Autodesk Inventor part; units mm, degrees
(part 13 of 15)
  arc A5791 (-48.3815, -55.2875) -> (-47.8186, -55.6125) centre (-48.1, -55.45) ccw
  arc A5792 (-47.8186, -55.6125) -> (-48.3815, -55.2875) centre (-48.1, -55.45) ccw
  arc A5793 (-48.3815, -55.2875) -> (-47.8186, -55.6125) centre (-48.1, -55.45) ccw
  arc A5794 (-49.6056, -55.4035) -> (-50.1685, -55.0785) centre (-49.887, -55.241) ccw
  arc A5795 (-50.1685, -55.0785) -> (-49.6056, -55.4035) centre (-49.887, -55.241) ccw
  arc A5796 (-49.6056, -55.4035) -> (-50.1685, -55.0785) centre (-49.887, -55.241) ccw
  arc A5797 (-50.1685, -55.0785) -> (-49.6056, -55.4035) centre (-49.887, -55.241) ccw
  arc A5798 (-51.2966, -54.7885) -> (-51.8595, -54.4635) centre (-51.578, -54.626) ccw
  arc A5799 (-51.8595, -54.4635) -> (-51.2966, -54.7885) centre (-51.578, -54.626) ccw
  arc A5800 (-51.2966, -54.7885) -> (-51.8595, -54.4635) centre (-51.578, -54.626) ccw
  arc A5801 (-51.8595, -54.4635) -> (-51.2966, -54.7885) centre (-51.578, -54.626) ccw
  arc A5802 (-52.8006, -53.7995) -> (-53.3635, -53.4745) centre (-53.082, -53.637) ccw
  arc A5803 (-53.3635, -53.4745) -> (-52.8006, -53.7995) centre (-53.082, -53.637) ccw
  arc A5804 (-52.8006, -53.7995) -> (-53.3635, -53.4745) centre (-53.082, -53.637) ccw
  arc A5805 (-53.3635, -53.4745) -> (-52.8006, -53.7995) centre (-53.082, -53.637) ccw
  arc A5806 (-54.0346, -52.4905) -> (-54.5975, -52.1655) centre (-54.316, -52.328) ccw
  arc A5807 (-54.5975, -52.1655) -> (-54.0346, -52.4905) centre (-54.316, -52.328) ccw
  arc A5808 (-54.0346, -52.4905) -> (-54.5975, -52.1655) centre (-54.316, -52.328) ccw
  arc A5809 (-54.5975, -52.1655) -> (-54.0346, -52.4905) centre (-54.316, -52.328) ccw
  arc A5810 (-54.9346, -50.9325) -> (-55.4975, -50.6075) centre (-55.216, -50.77) ccw
  arc A5811 (-55.4975, -50.6075) -> (-54.9346, -50.9325) centre (-55.216, -50.77) ccw
  arc A5812 (-54.9346, -50.9325) -> (-55.4975, -50.6075) centre (-55.216, -50.77) ccw
  arc A5813 (-55.4975, -50.6075) -> (-54.9346, -50.9325) centre (-55.216, -50.77) ccw
  arc A5814 (-55.4506, -49.2085) -> (-56.0135, -48.8835) centre (-55.732, -49.046) ccw
  arc A5815 (-56.0135, -48.8835) -> (-55.4506, -49.2085) centre (-55.732, -49.046) ccw
  arc A5816 (-55.4506, -49.2085) -> (-56.0135, -48.8835) centre (-55.732, -49.046) ccw
  arc A5817 (-56.0135, -48.8835) -> (-55.4506, -49.2085) centre (-55.732, -49.046) ccw
  arc A5818 (-55.5556, -47.4115) -> (-56.1185, -47.0865) centre (-55.837, -47.249) ccw
  arc A5819 (-56.1185, -47.0865) -> (-55.5556, -47.4115) centre (-55.837, -47.249) ccw
  arc A5820 (-55.5556, -47.4115) -> (-56.1185, -47.0865) centre (-55.837, -47.249) ccw
  arc A5821 (-56.1185, -47.0865) -> (-55.5556, -47.4115) centre (-55.837, -47.249) ccw
  arc A5822 (-55.2426, -45.6395) -> (-55.8055, -45.3145) centre (-55.524, -45.477) ccw
  arc A5823 (-55.8055, -45.3145) -> (-55.2426, -45.6395) centre (-55.524, -45.477) ccw
  arc A5824 (-55.2426, -45.6395) -> (-55.8055, -45.3145) centre (-55.524, -45.477) ccw
  arc A5825 (-55.8055, -45.3145) -> (-55.2426, -45.6395) centre (-55.524, -45.477) ccw
  arc A5826 (-54.5306, -43.9875) -> (-55.0935, -43.6625) centre (-54.812, -43.825) ccw
  arc A5827 (-55.0935, -43.6625) -> (-54.5306, -43.9875) centre (-54.812, -43.825) ccw
  arc A5828 (-54.5306, -43.9875) -> (-55.0935, -43.6625) centre (-54.812, -43.825) ccw
  arc A5829 (-55.0935, -43.6625) -> (-54.5306, -43.9875) centre (-54.812, -43.825) ccw
  arc A5830 (-53.4556, -42.5445) -> (-54.0185, -42.2195) centre (-53.737, -42.382) ccw
  arc A5831 (-54.0185, -42.2195) -> (-53.4556, -42.5445) centre (-53.737, -42.382) ccw
  arc A5832 (-53.4556, -42.5445) -> (-54.0185, -42.2195) centre (-53.737, -42.382) ccw
  arc A5833 (-54.0185, -42.2195) -> (-53.4556, -42.5445) centre (-53.737, -42.382) ccw
  arc A5834 (-52.0776, -41.3875) -> (-52.6405, -41.0625) centre (-52.359, -41.225) ccw
  arc A5835 (-52.6405, -41.0625) -> (-52.0776, -41.3875) centre (-52.359, -41.225) ccw
  arc A5836 (-52.0776, -41.3875) -> (-52.6405, -41.0625) centre (-52.359, -41.225) ccw
  arc A5837 (-52.6405, -41.0625) -> (-52.0776, -41.3875) centre (-52.359, -41.225) ccw
  arc A5838 (-50.4696, -40.5795) -> (-51.0325, -40.2545) centre (-50.751, -40.417) ccw
  arc A5839 (-51.0325, -40.2545) -> (-50.4696, -40.5795) centre (-50.751, -40.417) ccw
  arc A5840 (-50.4696, -40.5795) -> (-51.0325, -40.2545) centre (-50.751, -40.417) ccw
  arc A5841 (-51.0325, -40.2545) -> (-50.4696, -40.5795) centre (-50.751, -40.417) ccw
  arc A5842 (-48.7186, -40.1645) -> (-49.2815, -39.8395) centre (-49, -40.002) ccw
  arc A5843 (-49.2815, -39.8395) -> (-48.7186, -40.1645) centre (-49, -40.002) ccw
  arc A5844 (-48.7186, -40.1645) -> (-49.2815, -39.8395) centre (-49, -40.002) ccw
  arc A5845 (-49.2815, -39.8395) -> (-48.7186, -40.1645) centre (-49, -40.002) ccw
  arc A5846 (-46.8996, -42.0595) -> (-47.4625, -41.7345) centre (-47.181, -41.897) ccw
  arc A5847 (-47.4625, -41.7345) -> (-46.8996, -42.0595) centre (-47.181, -41.897) ccw
  arc A5848 (-46.8996, -42.0595) -> (-47.4625, -41.7345) centre (-47.181, -41.897) ccw
  arc A5849 (-47.4625, -41.7345) -> (-46.8996, -42.0595) centre (-47.181, -41.897) ccw
  arc A5850 (-45.1516, -42.6275) -> (-45.7145, -42.3025) centre (-45.433, -42.465) ccw
  arc A5851 (-45.7145, -42.3025) -> (-45.1516, -42.6275) centre (-45.433, -42.465) ccw
  arc A5852 (-45.1516, -42.6275) -> (-45.7145, -42.3025) centre (-45.433, -42.465) ccw
  arc A5853 (-45.7145, -42.3025) -> (-45.1516, -42.6275) centre (-45.433, -42.465) ccw
  arc A5854 (-43.6646, -43.7085) -> (-44.2275, -43.3835) centre (-43.946, -43.546) ccw
  arc A5855 (-44.2275, -43.3835) -> (-43.6646, -43.7085) centre (-43.946, -43.546) ccw
  arc A5856 (-43.6646, -43.7085) -> (-44.2275, -43.3835) centre (-43.946, -43.546) ccw
  arc A5857 (-44.2275, -43.3835) -> (-43.6646, -43.7085) centre (-43.946, -43.546) ccw
  arc A5858 (-42.5836, -45.1955) -> (-43.1465, -44.8705) centre (-42.865, -45.033) ccw
  arc A5859 (-43.1465, -44.8705) -> (-42.5836, -45.1955) centre (-42.865, -45.033) ccw
  arc A5860 (-42.5836, -45.1955) -> (-43.1465, -44.8705) centre (-42.865, -45.033) ccw
  arc A5861 (-43.1465, -44.8705) -> (-42.5836, -45.1955) centre (-42.865, -45.033) ccw
  arc A5862 (-42.0156, -46.9435) -> (-42.5785, -46.6185) centre (-42.297, -46.781) ccw
  arc A5863 (-42.5785, -46.6185) -> (-42.0156, -46.9435) centre (-42.297, -46.781) ccw
  arc A5864 (-42.0156, -46.9435) -> (-42.5785, -46.6185) centre (-42.297, -46.781) ccw
  arc A5865 (-42.5785, -46.6185) -> (-42.0156, -46.9435) centre (-42.297, -46.781) ccw
  arc A5866 (-42.0156, -48.7815) -> (-42.5785, -48.4565) centre (-42.297, -48.619) ccw
  arc A5867 (-42.5785, -48.4565) -> (-42.0156, -48.7815) centre (-42.297, -48.619) ccw
  arc A5868 (-42.0156, -48.7815) -> (-42.5785, -48.4565) centre (-42.297, -48.619) ccw
  arc A5869 (-42.5785, -48.4565) -> (-42.0156, -48.7815) centre (-42.297, -48.619) ccw
  arc A5870 (-42.5836, -50.5295) -> (-43.1465, -50.2045) centre (-42.865, -50.367) ccw
  arc A5871 (-43.1465, -50.2045) -> (-42.5836, -50.5295) centre (-42.865, -50.367) ccw
  arc A5872 (-42.5836, -50.5295) -> (-43.1465, -50.2045) centre (-42.865, -50.367) ccw
  arc A5873 (-43.1465, -50.2045) -> (-42.5836, -50.5295) centre (-42.865, -50.367) ccw
  arc A5874 (-43.6646, -52.0165) -> (-44.2275, -51.6915) centre (-43.946, -51.854) ccw
  arc A5875 (-44.2275, -51.6915) -> (-43.6646, -52.0165) centre (-43.946, -51.854) ccw
  arc A5876 (-43.6646, -52.0165) -> (-44.2275, -51.6915) centre (-43.946, -51.854) ccw
  arc A5877 (-44.2275, -51.6915) -> (-43.6646, -52.0165) centre (-43.946, -51.854) ccw
  arc A5878 (-45.1516, -53.0975) -> (-45.7145, -52.7725) centre (-45.433, -52.935) ccw
  arc A5879 (-45.7145, -52.7725) -> (-45.1516, -53.0975) centre (-45.433, -52.935) ccw
  arc A5880 (-45.1516, -53.0975) -> (-45.7145, -52.7725) centre (-45.433, -52.935) ccw
  arc A5881 (-45.7145, -52.7725) -> (-45.1516, -53.0975) centre (-45.433, -52.935) ccw
  arc A5882 (-46.8996, -53.6655) -> (-47.4625, -53.3405) centre (-47.181, -53.503) ccw
  arc A5883 (-47.4625, -53.3405) -> (-46.8996, -53.6655) centre (-47.181, -53.503) ccw
  arc A5884 (-46.8996, -53.6655) -> (-47.4625, -53.3405) centre (-47.181, -53.503) ccw
  arc A5885 (-47.4625, -53.3405) -> (-46.8996, -53.6655) centre (-47.181, -53.503) ccw
  arc A5886 (-48.7376, -53.6655) -> (-49.3005, -53.3405) centre (-49.019, -53.503) ccw
  arc A5887 (-49.3005, -53.3405) -> (-48.7376, -53.6655) centre (-49.019, -53.503) ccw
  arc A5888 (-48.7376, -53.6655) -> (-49.3005, -53.3405) centre (-49.019, -53.503) ccw
  arc A5889 (-49.3005, -53.3405) -> (-48.7376, -53.6655) centre (-49.019, -53.503) ccw
  arc A5890 (-50.4856, -53.0975) -> (-51.0485, -52.7725) centre (-50.767, -52.935) ccw
  arc A5891 (-51.0485, -52.7725) -> (-50.4856, -53.0975) centre (-50.767, -52.935) ccw
  arc A5892 (-50.4856, -53.0975) -> (-51.0485, -52.7725) centre (-50.767, -52.935) ccw
  arc A5893 (-51.0485, -52.7725) -> (-50.4856, -53.0975) centre (-50.767, -52.935) ccw
  arc A5894 (-51.9726, -52.0165) -> (-52.5355, -51.6915) centre (-52.254, -51.854) ccw
  arc A5895 (-52.5355, -51.6915) -> (-51.9726, -52.0165) centre (-52.254, -51.854) ccw
  arc A5896 (-51.9726, -52.0165) -> (-52.5355, -51.6915) centre (-52.254, -51.854) ccw
  arc A5897 (-52.5355, -51.6915) -> (-51.9726, -52.0165) centre (-52.254, -51.854) ccw
  arc A5898 (-53.0536, -50.5295) -> (-53.6165, -50.2045) centre (-53.335, -50.367) ccw
  arc A5899 (-53.6165, -50.2045) -> (-53.0536, -50.5295) centre (-53.335, -50.367) ccw
  arc A5900 (-53.0536, -50.5295) -> (-53.6165, -50.2045) centre (-53.335, -50.367) ccw
  arc A5901 (-53.6165, -50.2045) -> (-53.0536, -50.5295) centre (-53.335, -50.367) ccw
  arc A5902 (-53.6216, -48.7815) -> (-54.1845, -48.4565) centre (-53.903, -48.619) ccw
  arc A5903 (-54.1845, -48.4565) -> (-53.6216, -48.7815) centre (-53.903, -48.619) ccw
  arc A5904 (-53.6216, -48.7815) -> (-54.1845, -48.4565) centre (-53.903, -48.619) ccw
  arc A5905 (-54.1845, -48.4565) -> (-53.6216, -48.7815) centre (-53.903, -48.619) ccw
  arc A5906 (-53.6216, -46.9435) -> (-54.1845, -46.6185) centre (-53.903, -46.781) ccw
  arc A5907 (-54.1845, -46.6185) -> (-53.6216, -46.9435) centre (-53.903, -46.781) ccw
  arc A5908 (-53.6216, -46.9435) -> (-54.1845, -46.6185) centre (-53.903, -46.781) ccw
  arc A5909 (-54.1845, -46.6185) -> (-53.6216, -46.9435) centre (-53.903, -46.781) ccw
  arc A5910 (-53.0536, -45.1955) -> (-53.6165, -44.8705) centre (-53.335, -45.033) ccw
  arc A5911 (-53.6165, -44.8705) -> (-53.0536, -45.1955) centre (-53.335, -45.033) ccw
  arc A5912 (-53.0536, -45.1955) -> (-53.6165, -44.8705) centre (-53.335, -45.033) ccw
  arc A5913 (-53.6165, -44.8705) -> (-53.0536, -45.1955) centre (-53.335, -45.033) ccw
  arc A5914 (-51.9726, -43.7085) -> (-52.5355, -43.3835) centre (-52.254, -43.546) ccw
  arc A5915 (-52.5355, -43.3835) -> (-51.9726, -43.7085) centre (-52.254, -43.546) ccw
  arc A5916 (-51.9726, -43.7085) -> (-52.5355, -43.3835) centre (-52.254, -43.546) ccw
  arc A5917 (-52.5355, -43.3835) -> (-51.9726, -43.7085) centre (-52.254, -43.546) ccw
  arc A5918 (-50.4856, -42.6275) -> (-51.0485, -42.3025) centre (-50.767, -42.465) ccw
  arc A5919 (-51.0485, -42.3025) -> (-50.4856, -42.6275) centre (-50.767, -42.465) ccw
  arc A5920 (-50.4856, -42.6275) -> (-51.0485, -42.3025) centre (-50.767, -42.465) ccw
  arc A5921 (-51.0485, -42.3025) -> (-50.4856, -42.6275) centre (-50.767, -42.465) ccw
  arc A5922 (-48.7376, -42.0595) -> (-49.3005, -41.7345) centre (-49.019, -41.897) ccw
  arc A5923 (-49.3005, -41.7345) -> (-48.7376, -42.0595) centre (-49.019, -41.897) ccw
  arc A5924 (-48.7376, -42.0595) -> (-49.3005, -41.7345) centre (-49.019, -41.897) ccw
  arc A5925 (-49.3005, -41.7345) -> (-48.7376, -42.0595) centre (-49.019, -41.897) ccw
  arc A5926 (-46.8616, -43.9785) -> (-47.4245, -43.6535) centre (-47.143, -43.816) ccw
  arc A5927 (-47.4245, -43.6535) -> (-46.8616, -43.9785) centre (-47.143, -43.816) ccw
  arc A5928 (-46.8616, -43.9785) -> (-47.4245, -43.6535) centre (-47.143, -43.816) ccw
  arc A5929 (-47.4245, -43.6535) -> (-46.8616, -43.9785) centre (-47.143, -43.816) ccw
  arc A5930 (-45.1666, -44.8685) -> (-45.7295, -44.5435) centre (-45.448, -44.706) ccw
  arc A5931 (-45.7295, -44.5435) -> (-45.1666, -44.8685) centre (-45.448, -44.706) ccw
  arc A5932 (-45.1666, -44.8685) -> (-45.7295, -44.5435) centre (-45.448, -44.706) ccw
  arc A5933 (-45.7295, -44.5435) -> (-45.1666, -44.8685) centre (-45.448, -44.706) ccw
  arc A5934 (-44.0786, -46.4445) -> (-44.6415, -46.1195) centre (-44.36, -46.282) ccw
  arc A5935 (-44.6415, -46.1195) -> (-44.0786, -46.4445) centre (-44.36, -46.282) ccw
  arc A5936 (-44.0786, -46.4445) -> (-44.6415, -46.1195) centre (-44.36, -46.282) ccw
  arc A5937 (-44.6415, -46.1195) -> (-44.0786, -46.4445) centre (-44.36, -46.282) ccw
  arc A5938 (-43.8476, -48.3445) -> (-44.4105, -48.0195) centre (-44.129, -48.182) ccw
  arc A5939 (-44.4105, -48.0195) -> (-43.8476, -48.3445) centre (-44.129, -48.182) ccw
  arc A5940 (-43.8476, -48.3445) -> (-44.4105, -48.0195) centre (-44.129, -48.182) ccw
  arc A5941 (-44.4105, -48.0195) -> (-43.8476, -48.3445) centre (-44.129, -48.182) ccw
  arc A5942 (-44.5266, -50.1345) -> (-45.0895, -49.8095) centre (-44.808, -49.972) ccw
  arc A5943 (-45.0895, -49.8095) -> (-44.5266, -50.1345) centre (-44.808, -49.972) ccw
  arc A5944 (-44.5266, -50.1345) -> (-45.0895, -49.8095) centre (-44.808, -49.972) ccw
  arc A5945 (-45.0895, -49.8095) -> (-44.5266, -50.1345) centre (-44.808, -49.972) ccw
  arc A5946 (-45.9596, -51.4045) -> (-46.5225, -51.0795) centre (-46.241, -51.242) ccw
  arc A5947 (-46.5225, -51.0795) -> (-45.9596, -51.4045) centre (-46.241, -51.242) ccw
  arc A5948 (-45.9596, -51.4045) -> (-46.5225, -51.0795) centre (-46.241, -51.242) ccw
  arc A5949 (-46.5225, -51.0795) -> (-45.9596, -51.4045) centre (-46.241, -51.242) ccw
  arc A5950 (-47.8186, -51.8625) -> (-48.3815, -51.5375) centre (-48.1, -51.7) ccw
  arc A5951 (-48.3815, -51.5375) -> (-47.8186, -51.8625) centre (-48.1, -51.7) ccw
  arc A5952 (-47.8186, -51.8625) -> (-48.3815, -51.5375) centre (-48.1, -51.7) ccw
  arc A5953 (-48.3815, -51.5375) -> (-47.8186, -51.8625) centre (-48.1, -51.7) ccw
  arc A5954 (-49.6776, -51.4045) -> (-50.2405, -51.0795) centre (-49.959, -51.242) ccw
  arc A5955 (-50.2405, -51.0795) -> (-49.6776, -51.4045) centre (-49.959, -51.242) ccw
  arc A5956 (-49.6776, -51.4045) -> (-50.2405, -51.0795) centre (-49.959, -51.242) ccw
  arc A5957 (-50.2405, -51.0795) -> (-49.6776, -51.4045) centre (-49.959, -51.242) ccw
  arc A5958 (-51.1106, -50.1345) -> (-51.6735, -49.8095) centre (-51.392, -49.972) ccw
  arc A5959 (-51.6735, -49.8095) -> (-51.1106, -50.1345) centre (-51.392, -49.972) ccw
  arc A5960 (-51.1106, -50.1345) -> (-51.6735, -49.8095) centre (-51.392, -49.972) ccw
  arc A5961 (-51.6735, -49.8095) -> (-51.1106, -50.1345) centre (-51.392, -49.972) ccw
  arc A5962 (-51.7896, -48.3445) -> (-52.3525, -48.0195) centre (-52.071, -48.182) ccw
  arc A5963 (-52.3525, -48.0195) -> (-51.7896, -48.3445) centre (-52.071, -48.182) ccw
  arc A5964 (-51.7896, -48.3445) -> (-52.3525, -48.0195) centre (-52.071, -48.182) ccw
  arc A5965 (-52.3525, -48.0195) -> (-51.7896, -48.3445) centre (-52.071, -48.182) ccw
  arc A5966 (-51.5586, -46.4445) -> (-52.1215, -46.1195) centre (-51.84, -46.282) ccw
  arc A5967 (-52.1215, -46.1195) -> (-51.5586, -46.4445) centre (-51.84, -46.282) ccw
  arc A5968 (-51.5586, -46.4445) -> (-52.1215, -46.1195) centre (-51.84, -46.282) ccw
  arc A5969 (-52.1215, -46.1195) -> (-51.5586, -46.4445) centre (-51.84, -46.282) ccw
  arc A5970 (-50.4706, -44.8685) -> (-51.0335, -44.5435) centre (-50.752, -44.706) ccw
  arc A5971 (-51.0335, -44.5435) -> (-50.4706, -44.8685) centre (-50.752, -44.706) ccw
  arc A5972 (-50.4706, -44.8685) -> (-51.0335, -44.5435) centre (-50.752, -44.706) ccw
  arc A5973 (-51.0335, -44.5435) -> (-50.4706, -44.8685) centre (-50.752, -44.706) ccw
  arc A5974 (-48.7756, -43.9785) -> (-49.3385, -43.6535) centre (-49.057, -43.816) ccw
  arc A5975 (-49.3385, -43.6535) -> (-48.7756, -43.9785) centre (-49.057, -43.816) ccw
  arc A5976 (-48.7756, -43.9785) -> (-49.3385, -43.6535) centre (-49.057, -43.816) ccw
  arc A5977 (-49.3385, -43.6535) -> (-48.7756, -43.9785) centre (-49.057, -43.816) ccw
  arc A5978 (-47.8186, -45.7375) -> (-48.3815, -45.4125) centre (-48.1, -45.575) ccw
  arc A5979 (-48.3815, -45.4125) -> (-47.8186, -45.7375) centre (-48.1, -45.575) ccw
  arc A5980 (-47.8186, -45.7375) -> (-48.3815, -45.4125) centre (-48.1, -45.575) ccw
  arc A5981 (-48.3815, -45.4125) -> (-47.8186, -45.7375) centre (-48.1, -45.575) ccw
  arc A5982 (-46.1576, -46.5375) -> (-46.7205, -46.2125) centre (-46.439, -46.375) ccw
  arc A5983 (-46.7205, -46.2125) -> (-46.1576, -46.5375) centre (-46.439, -46.375) ccw
  arc A5984 (-46.1576, -46.5375) -> (-46.7205, -46.2125) centre (-46.439, -46.375) ccw
  arc A5985 (-46.7205, -46.2125) -> (-46.1576, -46.5375) centre (-46.439, -46.375) ccw
  arc A5986 (-45.7466, -48.3355) -> (-46.3095, -48.0105) centre (-46.028, -48.173) ccw
  arc A5987 (-46.3095, -48.0105) -> (-45.7466, -48.3355) centre (-46.028, -48.173) ccw
  arc A5988 (-45.7466, -48.3355) -> (-46.3095, -48.0105) centre (-46.028, -48.173) ccw
  arc A5989 (-46.3095, -48.0105) -> (-45.7466, -48.3355) centre (-46.028, -48.173) ccw
  arc A5990 (-46.8966, -49.7775) -> (-47.4595, -49.4525) centre (-47.178, -49.615) ccw
  arc A5991 (-47.4595, -49.4525) -> (-46.8966, -49.7775) centre (-47.178, -49.615) ccw
  arc A5992 (-46.8966, -49.7775) -> (-47.4595, -49.4525) centre (-47.178, -49.615) ccw
  arc A5993 (-47.4595, -49.4525) -> (-46.8966, -49.7775) centre (-47.178, -49.615) ccw
  arc A5994 (-48.7406, -49.7775) -> (-49.3035, -49.4525) centre (-49.022, -49.615) ccw
  arc A5995 (-49.3035, -49.4525) -> (-48.7406, -49.7775) centre (-49.022, -49.615) ccw
  arc A5996 (-48.7406, -49.7775) -> (-49.3035, -49.4525) centre (-49.022, -49.615) ccw
  arc A5997 (-49.3035, -49.4525) -> (-48.7406, -49.7775) centre (-49.022, -49.615) ccw
  arc A5998 (-49.8906, -48.3355) -> (-50.4535, -48.0105) centre (-50.172, -48.173) ccw
  arc A5999 (-50.4535, -48.0105) -> (-49.8906, -48.3355) centre (-50.172, -48.173) ccw
  arc A6000 (-49.8906, -48.3355) -> (-50.4535, -48.0105) centre (-50.172, -48.173) ccw
  arc A6001 (-50.4535, -48.0105) -> (-49.8906, -48.3355) centre (-50.172, -48.173) ccw
  arc A6002 (-49.4796, -46.5375) -> (-50.0425, -46.2125) centre (-49.761, -46.375) ccw
  arc A6003 (-50.0425, -46.2125) -> (-49.4796, -46.5375) centre (-49.761, -46.375) ccw
  arc A6004 (-49.4796, -46.5375) -> (-50.0425, -46.2125) centre (-49.761, -46.375) ccw
  arc A6005 (-50.0425, -46.2125) -> (-49.4796, -46.5375) centre (-49.761, -46.375) ccw
  arc A6006 (-47.8186, -47.8625) -> (-48.3815, -47.5375) centre (-48.1, -47.7) ccw
  arc A6007 (-48.3815, -47.5375) -> (-47.8186, -47.8625) centre (-48.1, -47.7) ccw
  arc A6008 (-47.8186, -47.8625) -> (-48.3815, -47.5375) centre (-48.1, -47.7) ccw
  arc A6009 (-48.3815, -47.5375) -> (-47.8186, -47.8625) centre (-48.1, -47.7) ccw
  arc A6010 (-39.5203, -56.1425) -> (-40.1698, -55.7675) centre (-39.845, -55.955) ccw
  arc A6011 (-40.1698, -55.7675) -> (-39.5203, -56.1425) centre (-39.845, -55.955) ccw
  arc A6012 (-39.5203, -56.1425) -> (-40.1698, -55.7675) centre (-39.845, -55.955) ccw
  arc A6013 (-40.1698, -55.7675) -> (-39.5203, -56.1425) centre (-39.845, -55.955) ccw
  arc A6014 (-56.0303, -56.1425) -> (-56.6798, -55.7675) centre (-56.355, -55.955) ccw
  arc A6015 (-56.6798, -55.7675) -> (-56.0303, -56.1425) centre (-56.355, -55.955) ccw
  arc A6016 (-56.0303, -56.1425) -> (-56.6798, -55.7675) centre (-56.355, -55.955) ccw
  arc A6017 (-56.6798, -55.7675) -> (-56.0303, -56.1425) centre (-56.355, -55.955) ccw
  arc A6018 (-56.0303, -39.6325) -> (-56.6798, -39.2575) centre (-56.355, -39.445) ccw
  arc A6019 (-56.6798, -39.2575) -> (-56.0303, -39.6325) centre (-56.355, -39.445) ccw
  arc A6020 (-56.0303, -39.6325) -> (-56.6798, -39.2575) centre (-56.355, -39.445) ccw
  arc A6021 (-56.6798, -39.2575) -> (-56.0303, -39.6325) centre (-56.355, -39.445) ccw
  arc A6022 (-39.5203, -39.6325) -> (-40.1698, -39.2575) centre (-39.845, -39.445) ccw
  arc A6023 (-40.1698, -39.2575) -> (-39.5203, -39.6325) centre (-39.845, -39.445) ccw
  arc A6024 (-39.5203, -39.6325) -> (-40.1698, -39.2575) centre (-39.845, -39.445) ccw
  arc A6025 (-40.1698, -39.2575) -> (-39.5203, -39.6325) centre (-39.845, -39.445) ccw
  arc A6026 (-25.4554, 58.14) -> (-26.5086, 58.14) centre (-25.982, 58.14) ccw
  arc A6027 (-26.5086, 58.14) -> (-25.4554, 58.14) centre (-25.982, 58.14) ccw
  arc A6028 (-25.4554, 58.14) -> (-26.5086, 58.14) centre (-25.982, 58.14) ccw
  arc A6029 (-26.5086, 58.14) -> (-25.4554, 58.14) centre (-25.982, 58.14) ccw
  arc A6030 (-20.3754, 58.14) -> (-21.4286, 58.14) centre (-20.902, 58.14) ccw
  arc A6031 (-21.4286, 58.14) -> (-20.3754, 58.14) centre (-20.902, 58.14) ccw
  arc A6032 (-20.3754, 58.14) -> (-21.4286, 58.14) centre (-20.902, 58.14) ccw
  arc A6033 (-21.4286, 58.14) -> (-20.3754, 58.14) centre (-20.902, 58.14) ccw
  arc A6034 (-20.3754, 53.06) -> (-21.4286, 53.06) centre (-20.902, 53.06) ccw
  arc A6035 (-21.4286, 53.06) -> (-20.3754, 53.06) centre (-20.902, 53.06) ccw
  arc A6036 (-20.3754, 53.06) -> (-21.4286, 53.06) centre (-20.902, 53.06) ccw
  arc A6037 (-21.4286, 53.06) -> (-20.3754, 53.06) centre (-20.902, 53.06) ccw
  arc A6038 (-25.4554, 53.06) -> (-26.5086, 53.06) centre (-25.982, 53.06) ccw
  arc A6039 (-26.5086, 53.06) -> (-25.4554, 53.06) centre (-25.982, 53.06) ccw
  arc A6040 (-25.4554, 53.06) -> (-26.5086, 53.06) centre (-25.982, 53.06) ccw
  arc A6041 (-26.5086, 53.06) -> (-25.4554, 53.06) centre (-25.982, 53.06) ccw
  arc A6042 (-22.9654, 55.6) -> (-23.9186, 55.6) centre (-23.442, 55.6) ccw
  arc A6043 (-23.9186, 55.6) -> (-22.9654, 55.6) centre (-23.442, 55.6) ccw
  arc A6044 (-22.9654, 55.6) -> (-23.9186, 55.6) centre (-23.442, 55.6) ccw
  arc A6045 (-23.9186, 55.6) -> (-22.9654, 55.6) centre (-23.442, 55.6) ccw
  line L2695 (-34.75, -39.5) -> (-33.75, -39.5)
  line L2696 (-33.75, -39.5) -> (-33.75, -38.5)
  line L2697 (-33.75, -38.5) -> (-34.75, -38.5)
  line L2698 (-34.75, -38.5) -> (-34.75, -39.5)
  line L2699 (-34.75, -56.7) -> (-33.75, -56.7)
  line L2700 (-33.75, -56.7) -> (-33.75, -55.7)
  line L2701 (-33.75, -55.7) -> (-34.75, -55.7)
  line L2702 (-34.75, -55.7) -> (-34.75, -56.7)
  point P0 (0, 0)
  point P1 (-57.9, -58.1)
  point P2 (-11.4, 48.7)
  point P3 (-13.2, 49.3)
  point P4 (-7.2, -84.7)
  point P5 (-15.5, -89)
  point P6 (-11.9, -96.4)
  point P7 (-17.3, -99.6)
  point P8 (-17.8, -104.1)
  point P9 (-17.3, -100.6)
  point P10 (-17.3, -101.6)
  point P11 (-10.4, -98.6)
  point P12 (-9, -101.3)
  point P13 (-10.4, -101.3)
  point P14 (-16.6, -107.9)
  point P15 (-15.3, -108.4)
  point P16 (10.9, -76.6)
  point P17 (10.6, -79.7)
  point P18 (8.8, -76.6)
  point P19 (10.6, -84.5)
  point P20 (13, -76.6)
  point P21 (14.4, -76.6)
  point P22 (15.8, -76.6)
  point P23 (-17.4, 37.7)
  point P24 (-22, -4.8)
  point P25 (18.1, -52.2)
  point P26 (-19.5, 39.3)
  point P27 (-20, 6.2)
  point P28 (-6, 7.2)
  point P29 (20.4, -111.8)
  point P30 (20.4, -115.2)
  point P31 (14.2, -106.4)
  point P32 (8.4, -108.6)
  point P33 (8.9, -107.1)
  point P34 (-7.4, -106.6)
  point P35 (12.7, -98.5)
  point P36 (12.7, -102.8)
  point P37 (11.5, -105.4)
  point P38 (13.2, -105.3)
  point P39 (-5.9, -108.1)
  point P40 (-4.4, -108.6)
  point P41 (15.2, -101.3)
  point P42 (15.2, -103.3)
  point P43 (-7.8, 44.5)
  point P44 (-10.6, 43.8)
  point P45 (-5.1, 41.2)
  point P46 (-7.7, 40)
  point P47 (-10.1, 38.2)
  point P48 (-2.7, 45.4)
  point P49 (1.4, -89.7)
  point P50 (-0.9, -90)
  point P51 (1.4, -91.4)
  point P52 (-13.5, 9.7)
  point P53 (-6, 8.7)
  point P54 (-8.7, 19.7)
  point P55 (-11.1, 19.2)
  point P56 (-14, 12.2)
  point P57 (-20, 3.2)
  point P58 (-10, 14.2)
  point P59 (-6.5, 4.2)
  point P60 (-15.5, -5.8)
  point P61 (-12, 12.2)
  point P62 (-7.5, 4.2)
  point P63 (-11.5, -9.8)
  point P64 (-13.5, -5.8)
  point P65 (-2.5, 4.2)
  point P66 (-9.5, 6.2)
  point P67 (2.5, 7.2)
  point P68 (-3, 12.7)
  point P69 (-16, 16.7)
  point P70 (-18, 0.7)
  point P71 (6.5, 12.2)
  point P72 (-17, 6.7)
  point P73 (-3, 11.7)
  point P74 (-19, 17.7)
  point P75 (-17.5, 13.2)
  point P76 (-15.5, 9.2)
  point P77 (4.5, 14.2)
  point P78 (-2.5, 8.2)
  point P79 (-17, 4.7)
  point P80 (-11, 4.2)
  point P81 (-6.8, 14.7)
  point P82 (-7, 12.7)
  point P83 (-10.5, 10.7)
  point P84 (-8.2, 14.7)
  point P85 (-18.6, 9.6)
  point P86 (-23, 10.2)
  point P87 (-3, -3.3)
  point P88 (-3, -6.3)
  point P89 (-14.7, 19.2)
  point P90 (-3, -2.3)
  point P91 (0, -1.3)
  point P92 (-16.5, 19.2)
  point P93 (-23, -9.9)
  point P94 (1.5, -3.8)
  point P95 (-5, -2.3)
  point P96 (-0.5, -3.8)
  point P97 (-12.9, 19.2)
  point P98 (-1.5, -2.8)
  point P99 (1.5, 0.2)
  point P100 (-2, -0.3)
  point P101 (-4, -10.3)
  point P102 (-6.5, -0.8)
  point P103 (-5, -6.3)
  point P104 (-23, 1.2)
  point P105 (-19.5, -0.8)
  point P106 (5.5, -5.8)
  point P107 (-23, 6.6)
  point P108 (21.6, -22.8)
  point P109 (23.4, -22.8)
  point P110 (-11, -0.3)
  point P111 (-23, 8.4)
  point P112 (2, 5.7)
  point P113 (-23, 3)
  point P114 (-23, 4.8)
  point P115 (-23, -0.6)
  point P116 (-4, -0.3)
  point P117 (-4.5, 1.2)
  point P118 (-17.5, 2.2)
  point P119 (-23.2, -22.9)
  point P120 (19.9, 20.7)
  point P121 (17.7, 20.7)
  point P122 (23.9, 16.7)
  point P123 (19.9, 10.3)
  point P124 (17.7, 10.3)
  point P125 (23.9, 6.3)
  point P126 (13.7, 12.7)
  point P127 (15.7, 12.7)
  point P128 (13.7, 20.7)
  point P129 (13.7, 2.3)
  point P130 (15.7, 2.3)
  point P131 (13.7, 10.3)
  point P132 (15.7, 20.7)
  point P133 (15.7, 16.7)
  point P134 (23.9, 12.7)
  point P135 (15.7, 10.3)
  point P136 (15.7, 6.2)
  point P137 (23.9, 2.3)
  point P138 (19.9, 12.7)
  point P139 (13.7, 16.7)
  point P140 (21.9, 20.7)
  point P141 (19.9, 2.3)
  point P142 (13.7, 6.2)
  point P143 (21.9, 10.3)
  point P144 (23.9, 20.7)
  point P145 (19.7, 16.7)
  point P146 (23.9, 10.3)
  point P147 (19.7, 6.2)
  point P148 (19.9, -0.1)
  point P149 (17.7, -0.1)
  point P150 (23.9, -4.1)
  point P151 (19.9, -10.5)
  point P152 (17.7, -10.5)
  point P153 (23.9, -14.5)
  point P154 (13.7, -8.1)
  point P155 (15.7, -8.1)
  point P156 (13.7, -0.1)
  point P157 (13.7, -18.5)
  point P158 (15.7, -18.5)
  point P159 (13.7, -10.5)
  point P160 (15.7, -0.1)
  point P161 (15.9, -4.1)
  point P162 (23.9, -8.1)
  point P163 (15.7, -10.5)
  point P164 (15.7, -14.5)
  point P165 (23.9, -18.5)
  point P166 (19.9, -8.1)
  point P167 (13.7, -4.1)
  point P168 (21.9, -0.1)
  point P169 (19.9, -18.5)
  point P170 (13.7, -14.5)
  point P171 (21.9, -10.5)
  point P172 (23.9, -0.1)
  point P173 (19.9, -4.1)
  point P174 (17.7, 21.7)
  point P175 (17.7, 16.7)
  point P176 (3.9, -23.3)
  point P177 (6.1, -23.3)
  point P178 (0.7, -19.3)
  point P179 (10.1, -15.3)
  point P180 (8.1, -15.3)
  point P181 (10.1, -23.3)
  point P182 (8.1, -23.3)
  point P183 (9.9, -18.8)
  point P184 (-0.1, -15.3)
  point P185 (3.9, -15.3)
  point P186 (9.9, -19.8)
  point P187 (1.9, -23.3)
  point P188 (-0.1, -23.3)
  point P189 (2.7, -19.3)
  point P190 (-10.6, -23.1)
  point P191 (-22.8, 41)
  point P192 (-18.6, 43)
  point P193 (-22.3, 39.5)
  point P194 (-21, 49.6)
  point P195 (-18.9, 41)
  point P196 (-22.8, 43)
  point P197 (-20.8, 43)
  point P198 (-21.8, 43)
  point P199 (-16.5, 40.3)
  constraints: 11994 point on circle, 6045 centre point, 5406 end point
sketch "BOTTOM - 20240902" plane through (0, 0, -1.742) normal (0, 0, 1) x (1, 0, 0)
  arc A0 (-26, -28) -> (-25.5, -28.5) centre (-25.5, -28) ccw construction
  line L0 (-22.8, -32.942) -> (-22.8, -37.5)
  arc A1 (-23.3, -38) -> (-22.8, -37.5) centre (-23.3, -37.5) ccw
  line L1 (-23.3, -38) -> (-29.8, -38)
  arc A2 (-30.3, -37.5) -> (-29.8, -38) centre (-29.8, -37.5) ccw
  line L2 (-30.3, -37.5) -> (-30.3, -31.2)
  arc A3 (-30.3, -31.2) -> (-30.8, -30.7) centre (-30.8, -31.2) ccw
  line L3 (-30.8, -30.7) -> (-76.8, -30.7)
  arc A4 (-76.8, -30.7) -> (-77.3, -31.2) centre (-76.8, -31.2) ccw
  line L4 (-77.3, -31.2) -> (-77.3, -49.2)
  arc A5 (-77.3, -49.2) -> (-75.3, -51.2) centre (-75.3, -49.2) ccw
  line L5 (-75.3, -51.2) -> (-71.048, -51.2)
  arc A6 (-65.048, -57.2) -> (-71.048, -51.2) centre (-71.048, -57.2) ccw
  line L6 (-65.048, -57.2) -> (-65.048, -62.7)
  arc A7 (-65.048, -62.7) -> (-63.048, -64.7) centre (-63.048, -62.7) ccw
  line L7 (-63.048, -64.7) -> (-30.8, -64.7)
  arc A8 (-30.8, -64.7) -> (-30.3, -64.2) centre (-30.8, -64.2) ccw
  line L8 (-30.3, -64.2) -> (-30.3, -59.8)
  arc A9 (-29.8, -59.3) -> (-30.3, -59.8) centre (-29.8, -59.8) ccw
  line L9 (-29.8, -59.3) -> (-23.3, -59.3)
  arc A10 (-22.8, -59.8) -> (-23.3, -59.3) centre (-23.3, -59.8) ccw
  line L10 (-22.8, -59.8) -> (-22.8, -62.458)
  arc A11 (-22.8, -62.458) -> (-22.3, -62.958) centre (-22.3, -62.458) ccw
  line L11 (-22.3, -62.958) -> (-16, -62.958)
  arc A12 (-16, -62.958) -> (-15.5, -62.458) centre (-16, -62.458) ccw
  line L12 (-15.5, -62.458) -> (-15.5, -60.4)
  arc A13 (25.5, -120.6) -> (26, -120.1) centre (25.5, -120.1) ccw
  line L13 (25.5, -120.6) -> (-25.5, -120.6)
  arc A14 (-26, -120.1) -> (-25.5, -120.6) centre (-25.5, -120.1) ccw
  line L14 (-26, -120.1) -> (-26, -66.6)
  arc A15 (-25.5, -66.1) -> (-26, -66.6) centre (-25.5, -66.6) ccw
  line L15 (-25.5, -66.1) -> (-16, -66.1)
  arc A16 (-15.5, -66.6) -> (-16, -66.1) centre (-16, -66.6) ccw
  line L16 (-15.5, -66.6) -> (-15.5, -72.9)
  arc A17 (-15.5, -72.9) -> (-15, -73.4) centre (-15, -72.9) ccw
  line L17 (-15, -59.9) -> (-13.5, -59.9)
  arc A18 (-13, -60.4) -> (-13.5, -59.9) centre (-13.5, -60.4) ccw
  line L18 (-13, -60.4) -> (-13, -72.9)
  arc A19 (-13.5, -73.4) -> (-13, -72.9) centre (-13.5, -72.9) ccw
  line L19 (-13.5, -73.4) -> (-15, -73.4)
  arc A20 (26, -73.9) -> (25.5, -73.4) centre (25.5, -73.9) ccw
  line L20 (26, -73.9) -> (26, -120.1)
  line L21 (7.4, 23.5) -> (7.4, 31.9)
  arc A21 (7.9, 32.4) -> (7.4, 31.9) centre (7.9, 31.9) ccw
  line L22 (7.9, 32.4) -> (12.55, 32.4)
  arc A22 (7.4, 23.5) -> (7.9, 23) centre (7.9, 23.5) ccw
  line L23 (7.9, 23) -> (25, 23)
  arc A23 (12.55, 32.4) -> (13.05, 32.9) centre (12.55, 32.9) ccw
  line L24 (13.05, 32.9) -> (13.05, 40.1)
  arc A24 (13.55, 40.6) -> (13.05, 40.1) centre (13.55, 40.1) ccw
  line L25 (13.55, 40.6) -> (36.8, 40.6)
  arc A25 (37.3, 40.1) -> (36.8, 40.6) centre (36.8, 40.1) ccw
  line L26 (37.3, 40.1) -> (37.3, 36)
  arc A26 (36.8, 35.5) -> (37.3, 36) centre (36.8, 36) ccw
  line L27 (36.8, 35.5) -> (34.4, 35.5)
  arc A27 (34.4, 35.5) -> (33.9, 35) centre (34.4, 35) ccw
  line L28 (33.9, 35) -> (33.9, 30.9)
  arc A28 (33.9, 30.9) -> (34.4, 30.4) centre (34.4, 30.9) ccw
  line L29 (38.9, 31.8) -> (38.9, 30.9)
  arc A29 (38.4, 30.4) -> (38.9, 30.9) centre (38.4, 30.9) ccw
  line L30 (38.4, 30.4) -> (34.4, 30.4)
  line L31 (77.3, 32.8) -> (77.3, 50.2)
  arc A30 (77.8, 50.7) -> (77.3, 50.2) centre (77.8, 50.2) ccw
  line L32 (77.8, 50.7) -> (79.8, 50.7)
  arc A31 (79.8, 50.7) -> (80.3, 51.2) centre (79.8, 51.2) ccw
  line L33 (80.3, 51.2) -> (80.3, 56.4)
  arc A32 (80.3, 56.4) -> (79.8, 56.9) centre (79.8, 56.4) ccw
  line L34 (79.8, 56.9) -> (58.9, 56.9)
  line L35 (54.4, 31.3) -> (57.9, 31.3)
  arc A33 (57.9, 31.3) -> (58.4, 31.8) centre (57.9, 31.8) ccw
  arc A34 (58.9, 32.3) -> (58.4, 31.8) centre (58.9, 31.8) ccw
  line L36 (58.9, 32.3) -> (76.8, 32.3)
  arc A35 (76.8, 32.3) -> (77.3, 32.8) centre (76.8, 32.8) ccw
  arc A36 (53.9, 31.8) -> (54.4, 31.3) centre (54.4, 31.8) ccw
  arc A37 (53.9, 31.8) -> (53.4, 32.3) centre (53.4, 31.8) ccw
  line L37 (53.4, 32.3) -> (39.4, 32.3)
  arc A38 (39.4, 32.3) -> (38.9, 31.8) centre (39.4, 31.8) ccw
  line L38 (36.8, 52) -> (13.55, 52)
  arc A39 (13.05, 52.5) -> (13.55, 52) centre (13.55, 52.5) ccw
  line L39 (13.05, 52.5) -> (13.05, 59.358)
  arc A40 (13.05, 59.358) -> (12.55, 59.858) centre (12.55, 59.358) ccw
  line L40 (12.55, 59.858) -> (-27.242, 59.858)
  arc A41 (36.8, 52) -> (37.3, 52.5) centre (36.8, 52.5) ccw
  line L41 (37.3, 52.5) -> (37.3, 53.2)
  arc A42 (-27.242, 59.858) -> (-27.742, 59.358) centre (-27.242, 59.358) ccw
  line L42 (-27.742, 59.358) -> (-27.742, 29.842)
  arc A43 (37.3, 53.2) -> (36.8, 53.7) centre (36.8, 53.2) ccw
  line L43 (36.8, 53.7) -> (34.4, 53.7)
  arc A44 (33.9, 54.2) -> (34.4, 53.7) centre (34.4, 54.2) ccw
  line L44 (33.9, 54.2) -> (33.9, 58.3)
  line L45 (-15, -26) -> (-13.5, -26)
  arc A45 (-13, -26.5) -> (-13.5, -26) centre (-13.5, -26.5) ccw
  line L46 (-13, -26.5) -> (-13, -35)
  arc A46 (-13.5, -35.5) -> (-13, -35) centre (-13.5, -35) ccw
  line L47 (-13.5, -35.5) -> (-15, -35.5)
  arc A47 (-15, -26) -> (-15.5, -26.5) centre (-15, -26.5) ccw
  line L48 (-15.5, -26.5) -> (-15.5, -28)
  arc A48 (-16, -28.5) -> (-15.5, -28) centre (-16, -28) ccw
  line L49 (-16, -28.5) -> (-25.5, -28.5)
  arc A49 (-26, -28) -> (-25.5, -28.5) centre (-25.5, -28) ccw
  line L50 (-26, -28) -> (-26, 25.5)
  arc A50 (-25.5, 26) -> (-26, 25.5) centre (-25.5, 25.5) ccw
  line L51 (-25.5, 26) -> (-20.6, 26)
  arc A51 (-20.1, 25.5) -> (-20.6, 26) centre (-20.6, 25.5) ccw
  line L52 (-20.1, 25.5) -> (-20.1, 23.5)
  arc A52 (-20.1, 23.5) -> (-19.6, 23) centre (-19.6, 23.5) ccw
  line L53 (-19.6, 32.4) -> (-18.3, 32.4)
  arc A53 (-17.8, 31.9) -> (-18.3, 32.4) centre (-18.3, 31.9) ccw
  line L54 (-17.8, 31.9) -> (-17.8, 23.5)
  arc A54 (-18.3, 23) -> (-17.8, 23.5) centre (-18.3, 23.5) ccw
  line L55 (-18.3, 23) -> (-19.6, 23)
  arc A55 (26, 22) -> (25, 23) centre (25, 22) ccw
  line L56 (26, 22) -> (26, -25.5)
  arc A56 (25.5, -26) -> (26, -25.5) centre (25.5, -25.5) ccw
  line L57 (-15.5, -35) -> (-15.5, -32.942)
  arc A57 (-15.5, -32.942) -> (-16, -32.442) centre (-16, -32.942) ccw
  line L58 (-16, -32.442) -> (-22.3, -32.442)
  arc A58 (-22.3, -32.442) -> (-22.8, -32.942) centre (-22.3, -32.942) ccw
  arc A59 (-15, -59.9) -> (-15.5, -60.4) centre (-15, -60.4) ccw
  arc A60 (25.5, -59.9) -> (26, -59.4) centre (25.5, -59.4) ccw
  line L59 (26, -59.4) -> (26, -36)
  arc A61 (26, -36) -> (25.5, -35.5) centre (25.5, -36) ccw
  arc A62 (-15.5, -35) -> (-15, -35.5) centre (-15, -35) ccw
  line L60 (25.5, -73.4) -> (25, -73.4)
  arc A63 (24.5, -72.9) -> (25, -73.4) centre (25, -72.9) ccw
  line L61 (24.5, -72.9) -> (24.5, -60.4)
  arc A64 (25, -59.9) -> (24.5, -60.4) centre (25, -60.4) ccw
  line L62 (25, -59.9) -> (25.5, -59.9)
  line L63 (24.5, -35) -> (24.5, -26.5)
  arc A65 (25, -26) -> (24.5, -26.5) centre (25, -26.5) ccw
  line L64 (25, -26) -> (25.5, -26)
  arc A66 (24.5, -35) -> (25, -35.5) centre (25, -35) ccw
  line L65 (25, -35.5) -> (25.5, -35.5)
  arc A67 (-27.742, 29.842) -> (-27.242, 29.342) centre (-27.242, 29.842) ccw
  line L66 (-27.242, 29.342) -> (-20.6, 29.342)
  arc A68 (-20.6, 29.342) -> (-20.1, 29.842) centre (-20.6, 29.842) ccw
  line L67 (-20.1, 29.842) -> (-20.1, 31.9)
  arc A69 (-19.6, 32.4) -> (-20.1, 31.9) centre (-19.6, 31.9) ccw
  arc A70 (34.4, 58.8) -> (33.9, 58.3) centre (34.4, 58.3) ccw
  arc A71 (58.4, 57.4) -> (58.9, 56.9) centre (58.9, 57.4) ccw
  arc A72 (58.4, 57.4) -> (57.9, 57.9) centre (57.9, 57.4) ccw
  line L68 (57.9, 57.9) -> (54.4, 57.9)
  arc A73 (54.4, 57.9) -> (53.9, 57.4) centre (54.4, 57.4) ccw
  arc A74 (53.4, 56.9) -> (53.9, 57.4) centre (53.4, 57.4) ccw
  line L69 (53.4, 56.9) -> (39.4, 56.9)
  arc A75 (38.9, 57.4) -> (39.4, 56.9) centre (39.4, 57.4) ccw
  line L70 (38.9, 57.4) -> (38.9, 58.3)
  arc A76 (38.9, 58.3) -> (38.4, 58.8) centre (38.4, 58.3) ccw
  line L71 (38.4, 58.8) -> (34.4, 58.8)
  circle A77 centre (-36.6, -61.378) radius 2
  circle A78 centre (-36.6, -34.022) radius 2
  circle A79 centre (-19.1, -36.062) radius 2
  circle A80 centre (-23.092, 32.962) radius 2
  circle A81 centre (-9.192, 56.238) radius 2
  circle A82 centre (36.4, 56.256) radius 2
  circle A83 centre (78.021, 53.178) radius 2
  circle A84 centre (36.4, 32.98) radius 2
  circle A85 centre (56.15, 55.6) radius 2
  circle A86 centre (56.15, 33.6) radius 2
  circle A87 centre (-19.1, -59.338) radius 2
  circle A88 centre (-67.2, -34.022) radius 2
  circle A89 centre (22.735, -49.7) radius 0.37
  circle A90 centre (22.735, -48.43) radius 0.37
  circle A91 centre (21.465, -52.24) radius 0.37
  circle A92 centre (73, 35.6) radius 1.5
  circle A93 centre (22.735, -52.24) radius 0.37
  circle A94 centre (21.465, -47.16) radius 0.37
  circle A95 centre (22.735, -47.16) radius 0.37
  circle A96 centre (73, 53.6) radius 1.5
  circle A97 centre (44.6, 53.6) radius 1.5
  circle A98 centre (23.035, -105.13) radius 0.37
  circle A99 centre (23.035, -106.4) radius 0.37
  circle A100 centre (23.035, -107.67) radius 0.37
  circle A101 centre (21.765, -105.13) radius 0.37
  circle A102 centre (44.6, 35.6) radius 1.5
  circle A103 centre (21.765, -106.4) radius 0.37
  circle A104 centre (21.765, -107.67) radius 0.37
  circle A105 centre (23.035, -103.86) radius 0.37
  circle A106 centre (21.765, -103.86) radius 0.37
  circle A107 centre (23.035, -108.94) radius 0.37
  circle A108 centre (21.765, -108.94) radius 0.37
  circle A109 centre (-11.095, -17.035) radius 0.37
  circle A110 centre (-12.365, -17.035) radius 0.37
  circle A111 centre (-11.095, -15.765) radius 0.37
  circle A112 centre (-12.365, -15.765) radius 0.37
  circle A113 centre (-9.825, -17.035) radius 0.37
  circle A114 centre (-9.825, -15.765) radius 0.37
  circle A115 centre (-14.905, -17.035) radius 0.37
  circle A116 centre (-16.175, -17.035) radius 0.37
  circle A117 centre (-14.905, -15.765) radius 0.37
  circle A118 centre (-16.175, -15.765) radius 0.37
  circle A119 centre (-13.635, -17.035) radius 0.37
  circle A120 centre (-13.635, -15.765) radius 0.37
  circle A121 centre (21.465, -50.97) radius 0.37
  circle A122 centre (21.465, -49.7) radius 0.37
  circle A123 centre (21.465, -48.43) radius 0.37
  circle A124 centre (22.735, -50.97) radius 0.37
  line L72 (41.116, 46.008) -> (39.084, 46.008)
  line L73 (-17.09, -75.3044) -> (-25.0275, -75.3044)
  line L74 (-25.0275, -75.3044) -> (-25.0275, -81.4956)
  line L75 (-25.0275, -81.4956) -> (-17.09, -81.4956)
  line L76 (-17.09, -81.4956) -> (-17.09, -75.3044)
  line L77 (39.084, 46.008) -> (39.084, 44.992)
  line L78 (-17.09, -81.8044) -> (-25.0275, -81.8044)
  line L79 (-25.0275, -81.8044) -> (-25.0275, -87.9956)
  line L80 (-25.0275, -87.9956) -> (-17.09, -87.9956)
  line L81 (-17.09, -87.9956) -> (-17.09, -81.8044)
  line L82 (39.084, 44.992) -> (41.116, 44.992)
  line L83 (-17.09, -88.0044) -> (-25.0275, -88.0044)
  line L84 (-25.0275, -88.0044) -> (-25.0275, -94.1956)
  line L85 (-25.0275, -94.1956) -> (-17.09, -94.1956)
  line L86 (-17.09, -94.1956) -> (-17.09, -88.0044)
  line L87 (41.116, 44.992) -> (41.116, 46.008)
  line L88 (-17.457, -99.7892) -> (-17.457, -94.8108)
  line L89 (-17.457, -94.8108) -> (-19.743, -94.8108)
  line L90 (-19.743, -94.8108) -> (-19.743, -99.7892)
  line L91 (-19.743, -99.7892) -> (-17.457, -99.7892)
  line L92 (41.116, 45.008) -> (39.084, 45.008)
  line L93 (-12.143, -94.8108) -> (-12.143, -99.7892)
  line L94 (-12.143, -99.7892) -> (-9.857, -99.7892)
  line L95 (-9.857, -99.7892) -> (-9.857, -94.8108)
  line L96 (-9.857, -94.8108) -> (-12.143, -94.8108)
  line L97 (39.084, 45.008) -> (39.084, 43.992)
  line L98 (1.413, -106.076) -> (-3.413, -106.076)
  line L99 (-3.413, -106.076) -> (-3.413, -109.124)
  line L100 (-3.413, -109.124) -> (1.413, -109.124)
  line L101 (1.413, -109.124) -> (1.413, -106.076)
  line L102 (39.084, 43.992) -> (41.116, 43.992)
  line L103 (1.413, -102.976) -> (-3.413, -102.976)
  line L104 (-3.413, -102.976) -> (-3.413, -106.024)
  line L105 (-3.413, -106.024) -> (1.413, -106.024)
  line L106 (1.413, -106.024) -> (1.413, -102.976)
  line L107 (41.116, 43.992) -> (41.116, 45.008)
  line L108 (-19.613, -106.724) -> (-14.787, -106.724)
  line L109 (-14.787, -106.724) -> (-14.787, -103.676)
  line L110 (-14.787, -103.676) -> (-19.613, -103.676)
  line L111 (-19.613, -103.676) -> (-19.613, -106.724)
  line L112 (11.616, 51.008) -> (9.584, 51.008)
  line L113 (-19.613, -103.524) -> (-14.787, -103.524)
  line L114 (-14.787, -103.524) -> (-14.787, -100.476)
  line L115 (-14.787, -100.476) -> (-19.613, -100.476)
  line L116 (-19.613, -100.476) -> (-19.613, -103.524)
  line L117 (9.584, 51.008) -> (9.584, 49.992)
  line L118 (-12.465, -110.197) -> (-12.465, -107.403)
  line L119 (-12.465, -107.403) -> (-13.735, -107.403)
  line L120 (-13.735, -107.403) -> (-13.735, -110.197)
  line L121 (-13.735, -110.197) -> (-12.465, -110.197)
  line L122 (9.584, 49.992) -> (11.616, 49.992)
  line L123 (-15.816, -108.408) -> (-13.784, -108.408)
  line L124 (-13.784, -108.408) -> (-13.784, -107.392)
  line L125 (-13.784, -107.392) -> (-15.816, -107.392)
  line L126 (-15.816, -107.392) -> (-15.816, -108.408)
  line L127 (11.616, 49.992) -> (11.616, 51.008)
  line L128 (-18.784, -110.792) -> (-20.816, -110.792)
  line L129 (-20.816, -110.792) -> (-20.816, -111.808)
  line L130 (-20.816, -111.808) -> (-18.784, -111.808)
  line L131 (-18.784, -111.808) -> (-18.784, -110.792)
  line L132 (11.616, 50.008) -> (9.584, 50.008)
  line L133 (-14.176, -117.113) -> (-14.176, -112.287)
  line L134 (-14.176, -112.287) -> (-17.224, -112.287)
  line L135 (-17.224, -112.287) -> (-17.224, -117.113)
  line L136 (-17.224, -117.113) -> (-14.176, -117.113)
  line L137 (9.584, 50.008) -> (9.584, 48.992)
  line L138 (16.7458, -84.589) -> (20.4542, -84.589)
  line L139 (20.4542, -84.589) -> (20.4542, -82.811)
  line L140 (20.4542, -82.811) -> (16.7458, -82.811)
  line L141 (16.7458, -82.811) -> (16.7458, -84.589)
  line L142 (9.584, 48.992) -> (11.616, 48.992)
  line L143 (10.411, -87.3458) -> (10.411, -91.0542)
  line L144 (10.411, -91.0542) -> (12.189, -91.0542)
  line L145 (12.189, -91.0542) -> (12.189, -87.3458)
  line L146 (12.189, -87.3458) -> (10.411, -87.3458)
  line L147 (11.616, 48.992) -> (11.616, 50.008)
  line L148 (16.7458, -82.589) -> (20.4542, -82.589)
  line L149 (20.4542, -82.589) -> (20.4542, -80.811)
  line L150 (20.4542, -80.811) -> (16.7458, -80.811)
  line L151 (16.7458, -80.811) -> (16.7458, -82.589)
  line L152 (11.616, 49.008) -> (9.584, 49.008)
  line L153 (15.035, -77.997) -> (15.035, -75.203)
  line L154 (15.035, -75.203) -> (13.765, -75.203)
  line L155 (13.765, -75.203) -> (13.765, -77.997)
  line L156 (13.765, -77.997) -> (15.035, -77.997)
  line L157 (9.584, 49.008) -> (9.584, 47.992)
  line L158 (7.0542, -82.811) -> (3.3458, -82.811)
  line L159 (3.3458, -82.811) -> (3.3458, -84.589)
  line L160 (3.3458, -84.589) -> (7.0542, -84.589)
  line L161 (7.0542, -84.589) -> (7.0542, -82.811)
  line L162 (9.584, 47.992) -> (11.616, 47.992)
  line L163 (16.435, -77.997) -> (16.435, -75.203)
  line L164 (16.435, -75.203) -> (15.165, -75.203)
  line L165 (15.165, -75.203) -> (15.165, -77.997)
  line L166 (15.165, -77.997) -> (16.435, -77.997)
  line L167 (11.616, 47.992) -> (11.616, 49.008)
  line L168 (9.435, -77.997) -> (9.435, -75.203)
  line L169 (9.435, -75.203) -> (8.165, -75.203)
  line L170 (8.165, -75.203) -> (8.165, -77.997)
  line L171 (8.165, -77.997) -> (9.435, -77.997)
  line L172 (9.616, 51.008) -> (7.584, 51.008)
  line L173 (7.0542, -80.811) -> (3.3458, -80.811)
  line L174 (3.3458, -80.811) -> (3.3458, -82.589)
  line L175 (3.3458, -82.589) -> (7.0542, -82.589)
  line L176 (7.0542, -82.589) -> (7.0542, -80.811)
  line L177 (7.584, 51.008) -> (7.584, 49.992)
  line L178 (13.635, -77.997) -> (13.635, -75.203)
  line L179 (13.635, -75.203) -> (12.365, -75.203)
  line L180 (12.365, -75.203) -> (12.365, -77.997)
  line L181 (12.365, -77.997) -> (13.635, -77.997)
  line L182 (7.584, 49.992) -> (9.616, 49.992)
  line L183 (12.235, -77.997) -> (12.235, -75.203)
  line L184 (12.235, -75.203) -> (10.965, -75.203)
  line L185 (10.965, -75.203) -> (10.965, -77.997)
  line L186 (10.965, -77.997) -> (12.235, -77.997)
  line L187 (9.616, 49.992) -> (9.616, 51.008)
  line L188 (10.116, -88.692) -> (8.084, -88.692)
  line L189 (8.084, -88.692) -> (8.084, -89.708)
  line L190 (8.084, -89.708) -> (10.116, -89.708)
  line L191 (10.116, -89.708) -> (10.116, -88.692)
  line L192 (9.584, 45.992) -> (11.616, 45.992)
  line L193 (6.084, -89.708) -> (8.116, -89.708)
  line L194 (8.116, -89.708) -> (8.116, -88.692)
  line L195 (8.116, -88.692) -> (6.084, -88.692)
  line L196 (6.084, -88.692) -> (6.084, -89.708)
  line L197 (11.616, 45.992) -> (11.616, 47.008)
  line L198 (4.792, -88.684) -> (4.792, -90.716)
  line L199 (4.792, -90.716) -> (5.808, -90.716)
  line L200 (5.808, -90.716) -> (5.808, -88.684)
  line L201 (5.808, -88.684) -> (4.792, -88.684)
  line L202 (11.616, 47.008) -> (9.584, 47.008)
  line L203 (10.835, -77.997) -> (10.835, -75.203)
  line L204 (10.835, -75.203) -> (9.565, -75.203)
  line L205 (9.565, -75.203) -> (9.565, -77.997)
  line L206 (9.565, -77.997) -> (10.835, -77.997)
  line L207 (9.584, 47.008) -> (9.584, 45.992)
  line L208 (20.124, -92.913) -> (20.124, -88.087)
  line L209 (20.124, -88.087) -> (17.076, -88.087)
  line L210 (17.076, -88.087) -> (17.076, -92.913)
  line L211 (17.076, -92.913) -> (20.124, -92.913)
  line L212 (11.616, 48.008) -> (9.584, 48.008)
  line L213 (-0.076, -87.713) -> (-0.076, -82.887)
  line L214 (-0.076, -82.887) -> (-3.124, -82.887)
  line L215 (-3.124, -82.887) -> (-3.124, -87.713)
  line L216 (-3.124, -87.713) -> (-0.076, -87.713)
  line L217 (9.584, 48.008) -> (9.584, 46.992)
  line L218 (17.113, -90.076) -> (12.287, -90.076)
  line L219 (12.287, -90.076) -> (12.287, -93.124)
  line L220 (12.287, -93.124) -> (17.113, -93.124)
  line L221 (17.113, -93.124) -> (17.113, -90.076)
  line L222 (9.584, 46.992) -> (11.616, 46.992)
  line L223 (3.024, -87.713) -> (3.024, -82.887)
  line L224 (3.024, -82.887) -> (-0.024, -82.887)
  line L225 (-0.024, -82.887) -> (-0.024, -87.713)
  line L226 (-0.024, -87.713) -> (3.024, -87.713)
  line L227 (11.616, 46.992) -> (11.616, 48.008)
  line L228 (17.176, -93.587) -> (17.176, -98.413)
  line L229 (17.176, -98.413) -> (20.224, -98.413)
  line L230 (20.224, -98.413) -> (20.224, -93.587)
  line L231 (20.224, -93.587) -> (17.176, -93.587)
  line L232 (-0.584, 50.908) -> (-2.616, 50.908)
  line L233 (17.113, -93.076) -> (12.287, -93.076)
  line L234 (12.287, -93.076) -> (12.287, -96.124)
  line L235 (12.287, -96.124) -> (17.113, -96.124)
  line L236 (17.113, -96.124) -> (17.113, -93.076)
  line L237 (-2.616, 50.908) -> (-2.616, 49.892)
  line L238 (-2, -53.6) -> (-0.4, -53.6)
  line L239 (-0.4, -53.6) -> (-0.4, -52.8)
  line L240 (-2, -52.8) -> (-2, -53.6)
  line L241 (-0.4, -52.8) -> (-2, -52.8)
  line L242 (-2.616, 49.892) -> (-0.584, 49.892)
  line L243 (18.8, -43.8) -> (18.8, -42.2)
  line L244 (18.8, -42.2) -> (18, -42.2)
  line L245 (18, -43.8) -> (18.8, -43.8)
  line L246 (18, -42.2) -> (18, -43.8)
  line L247 (-0.584, 49.892) -> (-0.584, 50.908)
  line L248 (2.2, -52.8) -> (0.6, -52.8)
  line L249 (0.6, -52.8) -> (0.6, -53.6)
  line L250 (2.2, -53.6) -> (2.2, -52.8)
  line L251 (0.6, -53.6) -> (2.2, -53.6)
  line L252 (1.616, 50.908) -> (-0.416, 50.908)
  line L253 (20.687, -80.424) -> (25.513, -80.424)
  line L254 (25.513, -80.424) -> (25.513, -77.376)
  line L255 (25.513, -77.376) -> (20.687, -77.376)
  line L256 (20.687, -77.376) -> (20.687, -80.424)
  line L257 (-0.416, 50.908) -> (-0.416, 49.892)
  line L258 (20.687, -77.324) -> (25.513, -77.324)
  line L259 (25.513, -77.324) -> (25.513, -74.276)
  line L260 (25.513, -74.276) -> (20.687, -74.276)
  line L261 (20.687, -74.276) -> (20.687, -77.324)
  line L262 (-0.416, 49.892) -> (1.616, 49.892)
  line L263 (-3.476, -79.913) -> (-3.476, -75.087)
  line L264 (-3.476, -75.087) -> (-6.524, -75.087)
  line L265 (-6.524, -75.087) -> (-6.524, -79.913)
  line L266 (-6.524, -79.913) -> (-3.476, -79.913)
  line L267 (1.616, 49.892) -> (1.616, 50.908)
  line L268 (-6.524, -79.787) -> (-6.524, -84.613)
  line L269 (-6.524, -84.613) -> (-3.476, -84.613)
  line L270 (-3.476, -84.613) -> (-3.476, -79.787)
  line L271 (-3.476, -79.787) -> (-6.524, -79.787)
  line L272 (-0.684, 58.708) -> (-2.716, 58.708)
  line L273 (2.724, -79.913) -> (2.724, -75.087)
  line L274 (2.724, -75.087) -> (-0.324, -75.087)
  line L275 (-0.324, -75.087) -> (-0.324, -79.913)
  line L276 (-0.324, -79.913) -> (2.724, -79.913)
  line L277 (-2.716, 58.708) -> (-2.716, 57.692)
  line L278 (-23.8, -19.9) -> (-25.4, -19.9)
  line L279 (-25.4, -19.9) -> (-25.4, -20.7)
  line L280 (-23.8, -20.7) -> (-23.8, -19.9)
  line L281 (-25.4, -20.7) -> (-23.8, -20.7)
  line L282 (-2.716, 57.692) -> (-0.684, 57.692)
  line L283 (-0.376, -79.913) -> (-0.376, -75.087)
  line L284 (-0.376, -75.087) -> (-3.424, -75.087)
  line L285 (-3.424, -75.087) -> (-3.424, -79.913)
  line L286 (-3.424, -79.913) -> (-0.376, -79.913)
  line L287 (-0.684, 57.692) -> (-0.684, 58.708)
  line L288 (20.687, -88.024) -> (25.513, -88.024)
  line L289 (25.513, -88.024) -> (25.513, -84.976)
  line L290 (25.513, -84.976) -> (20.687, -84.976)
  line L291 (20.687, -84.976) -> (20.687, -88.024)
  line L292 (3.492, 51.416) -> (3.492, 49.384)
  line L293 (20.687, -91.124) -> (25.513, -91.124)
  line L294 (25.513, -91.124) -> (25.513, -88.076)
  line L295 (25.513, -88.076) -> (20.687, -88.076)
  line L296 (20.687, -88.076) -> (20.687, -91.124)
  line L297 (3.492, 49.384) -> (4.508, 49.384)
  line L298 (20.687, -94.124) -> (25.513, -94.124)
  line L299 (25.513, -94.124) -> (25.513, -91.076)
  line L300 (25.513, -91.076) -> (20.687, -91.076)
  line L301 (20.687, -91.076) -> (20.687, -94.124)
  line L302 (4.508, 49.384) -> (4.508, 51.416)
  line L303 (20.687, -97.124) -> (25.513, -97.124)
  line L304 (25.513, -97.124) -> (25.513, -94.076)
  line L305 (25.513, -94.076) -> (20.687, -94.076)
  line L306 (20.687, -94.076) -> (20.687, -97.124)
  line L307 (4.508, 51.416) -> (3.492, 51.416)
  line L308 (16.308, -116.316) -> (16.308, -114.284)
  line L309 (16.308, -114.284) -> (15.292, -114.284)